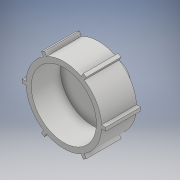
# Autodesk Inventor part: CamCap_holder
Saved by Autodesk Inventor 2018 (Build 220112000, 112)
## iProperties
Created: 2018-07-02
Part Number: CamCap_holder
Material: 一般
Document SubType Name: Modeling
Designer: izumi
Density: 1 g/cm^3
Appearance: 既定
Author: izumi
Autodesk Inventor part; units mm, degrees
ref_plane "YZ Plane" through (0, 0, 0) normal (1, 0, 0) x (0, 1, 0)
ref_plane "XZ Plane" through (0, 0, 0) normal (0, 1, 0) x (-1, 0, 0)
ref_plane "XY Plane" through (0, 0, 0) normal (0, 0, 1) x (1, 0, 0)
sketch "スケッチ1" plane through (0, 0, 0) normal (0, 1, 0) x (-1, 0, 0)
  circle A0 centre (0, 0) radius 6.5
  line L0 (0, 0) -> (0, -6.5) construction
  line L1 (3.5063, -5.4732) -> (2.9867, -5.7732)
  line L2 (2.9867, -5.7732) -> (3.3402, -6.3854)
  line L3 (3.3402, -6.3854) -> (3.8598, -6.0854)
  line L4 (3.8598, -6.0854) -> (3.5063, -5.4732)
  line L5 (0, 0) -> (3.6, -6.2354) construction
  line L6 (6.4931, 0.3) -> (6.4931, -0.3)
  line L7 (6.4931, -0.3) -> (7.2, -0.3)
  line L8 (7.2, -0.3) -> (7.2, 0.3)
  line L9 (7.2, 0.3) -> (6.4931, 0.3)
  line L10 (0, 0) -> (7.2, 0) construction
  line L11 (2.9867, 5.7732) -> (3.5063, 5.4732)
  line L12 (3.5063, 5.4732) -> (3.8598, 6.0854)
  line L13 (3.8598, 6.0854) -> (3.3402, 6.3854)
  line L14 (3.3402, 6.3854) -> (2.9867, 5.7732)
  line L15 (0, 0) -> (3.6, 6.2354) construction
  line L16 (-3.5063, 5.4732) -> (-2.9867, 5.7732)
  line L17 (-2.9867, 5.7732) -> (-3.3402, 6.3854)
  line L18 (-3.3402, 6.3854) -> (-3.8598, 6.0854)
  line L19 (-3.8598, 6.0854) -> (-3.5063, 5.4732)
  line L20 (0, 0) -> (-3.6, 6.2354) construction
  line L21 (-6.4931, -0.3) -> (-6.4931, 0.3)
  line L22 (0, 0) -> (-7.2, 0) construction
  line L23 (-6.4931, 0.3) -> (-7.2, 0.3)
  line L24 (-7.2, -0.3) -> (-6.4931, -0.3)
  line L25 (-7.2, 0.3) -> (-7.2, -0.3)
  line L26 (0, 0) -> (-3.6, -6.2354) construction
  line L27 (-2.9867, -5.7732) -> (-3.5063, -5.4732)
  line L28 (-3.5063, -5.4732) -> (-3.8598, -6.0854)
  line L29 (-3.8598, -6.0854) -> (-3.3402, -6.3854)
  line L30 (-3.3402, -6.3854) -> (-2.9867, -5.7732)
  dimension "d0" = 13
  dimension "d3" = 30
  dimension "d4" = 7.2
  dimension "d6" = 0.6
  dimension "d7" = 7.2
  dimension "d8" = 0.6
  dimension "d9" = 90
  dimension "d10" = 7.2
  dimension "d11" = 0.6
  dimension "d12" = 150
  dimension "d13" = 7.2
  dimension "d14" = 0.6
  dimension "d15" = 7.2
  dimension "d16" = 0.6
  dimension "d17" = 7.2
  dimension "d18" = 0.6
  dimension "d19" = 30
  dimension "d20" = 90
  dimension "d21" = 150
  constraints: 62 end point, 12 parallel, 12 perpendicular, 6 midpoint, 1 coincident, 1 vertical, 9 other
  measures "d3" angle of L0 L5
  measures "d4" distance of L0.start L5.end
  measures "d6" distance between parallel lines of L2 L4
  measures "d7" distance of L0.start L10.end
  measures "d8" distance between parallel lines of L7 L9
  measures "d9" angle of L10 L0
  measures "d10" distance of L0.start L15.end
  measures "d11" distance between parallel lines of L12 L14
  measures "d12" angle of L15 L0
  measures "d13" distance of L0.start L20.end
  measures "d14" distance between parallel lines of L17 L19
  measures "d15" distance of L0.start L22.end
  measures "d16" distance between parallel lines of L23 L24
  measures "d17" distance of L0.start L26.end
  measures "d18" distance between parallel lines of L28 L30
  measures "d19" angle of L26 L0
  measures "d20" angle of L0 L22
  measures "d21" angle of L20 L0
extrude "押し出し1" add sketch "スケッチ1" along normal blind 6
sketch "スケッチ2" plane through (0, 6, 0) normal (0, 1, 0) x (1, 0, 0)
  circle A0 centre (0, 0) radius 2.5
  dimension "d24" = 5
  constraints: 1 centre point, 1 coincident
  measures "d24" diameter of A0
extrude "押し出し2" add sketch "スケッチ2" along normal blind 3
sketch "スケッチ3" plane through (0, 9, 0) normal (0, 1, 0) x (1, 0, 0)
  point P0 (0, 0)
  point P1 (0, 0)
  constraints: 1 coincident
hole "穴1" at (0, 9, 0) direction (0, -1, 0) diameter 2.8 end through all
sketch "スケッチ4" plane through (0, 0, 0) normal (0, -1, 0) x (1, 0, 0)
  circle A0 centre (0, 0) radius 5.6
  dimension "d34" = 11.2
  constraints: 1 centre point, 1 coincident
  measures "d34" diameter of A0
extrude "押し出し3" cut sketch "スケッチ4" against normal blind 5
